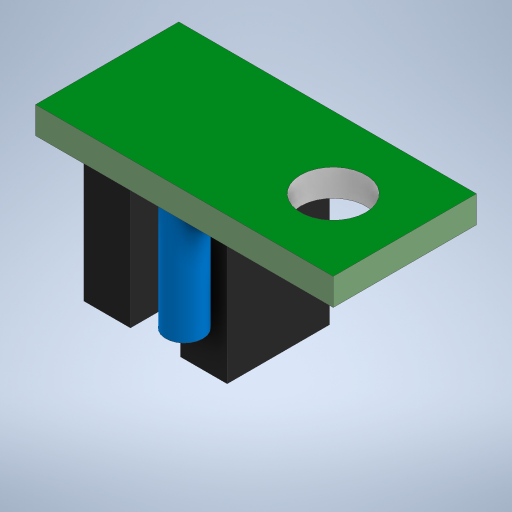
# Autodesk Inventor part: qre_module
Saved by Autodesk Inventor 2024 (Build 280153000, 153)
## iProperties
Created: 2023-11-08
Part Number: qre_module
Material: Všeobecné
Document SubType Name: Modeling
Designer: Simak
Density: 1 g/cm^3
Appearance: Výchozí
Author: Simak
Autodesk Inventor part; units mm, degrees
ref_plane "YZ Plane" through (0, 0, 0) normal (1, 0, 0) x (0, 1, 0)
ref_plane "XZ Plane" through (0, 0, 0) normal (0, 1, 0) x (-1, 0, 0)
ref_plane "XY Plane" through (0, 0, 0) normal (0, 0, 1) x (1, 0, 0)
sketch "Náčrt1" plane through (0, 0, 0) normal (0, 1, 0) x (-1, 0, 0)
  line L0 (8, -3.85) -> (-8, -3.85)
  line L1 (-8, -3.85) -> (-8, 3.85)
  line L2 (-8, 3.85) -> (8, 3.85)
  line L3 (8, 3.85) -> (8, -3.85)
  line L4 (8, -3.85) -> (0, 0) construction
  line L5 (8, 3.85) -> (0, 0) construction
  line L6 (-8, -3.85) -> (0, 0) construction
  dimension "d0" = 16
  dimension "d1" = 7.7
  constraints: 14 end point, 2 equal length, 2 parallel, 1 horizontal, 1 perpendicular
  measures "d0" distance of L0.start L0.end
  measures "d1" distance of L0.end L1.end
extrude "Vysunutí1" add sketch "Náčrt1" along normal blind 1.45
sketch "Náčrt2" plane through (0, 0, 0) normal (0, -1, 0) x (1, 0, 0)
  line L0 (0.2, 1.75) -> (-2.3, 1.75)
  line L1 (-2.3, 1.75) -> (-2.3, -3.75)
  line L2 (-2.3, -3.75) -> (0.2, -3.75)
  line L3 (0.2, -3.75) -> (0.2, 1.75)
  line L4 (-5, 1.75) -> (-7.5, 1.75)
  line L5 (-7.5, 1.75) -> (-7.5, -3.75)
  line L6 (-7.5, -3.75) -> (-5, -3.75)
  line L7 (-5, -3.75) -> (-5, 1.75)
  line L8 (-8, -3.85) -> (-8, 3.85) projected
  line L9 (-2.3, 1.75) -> (-5, 1.75) construction
  circle A0 centre (-3.65, -2.45) radius 1
  circle A1 centre (-1.05, 2.8) radius 1
  line L10 (-1.05, 1.75) -> (-1.05, 2.8) construction
  line L11 (-1.05, 2.8) -> (-1.05, 3.85) construction
  line L12 (-2.3, -2.45) -> (-3.65, -2.45) construction
  line L13 (-3.65, -2.45) -> (-5, -2.45) construction
  line L14 (-3.65, 1.75) -> (-3.65, 0.35) construction
  line L15 (-3.65, 0.35) -> (-3.65, -1.05) construction
  line L16 (-3.65, -1.05) -> (-3.65, -2.45) construction
  line L17 (-3.65, -3.85) -> (-3.65, -2.45) construction
  point P0 (0, 0)
  dimension "d4" = 2.5
  dimension "d5" = 5.5
  dimension "d6" = 0.5
  dimension "d7" = 2
  dimension "d8" = 2.7
  dimension "d15" = 0.1
  constraints: 34 end point, 8 point on line, 6 collinear, 5 equal length, 3 horizontal, 3 perpendicular, 2 centre point, 2 horizontal alignment, 2 midpoint, 2 vertical, 1 equal radius
  measures "d4" distance of L0.start L0.end
  measures "d5" distance of L2.end L0.start
  measures "d6" distance between parallel lines of L5 L8
  measures "d7" diameter of A0
  measures "d8" distance of L0.end L4.start
  measures "d15" vertical distance of L8.start L5.end
extrude "Vysunutí2" add sketch "Náčrt2" along normal blind 8.5 contours L3 L2 L1 L0 | L7 L6 L5 L4
extrude "Vysunutí3" add sketch "Náčrt2" along normal blind 6 contours A0 | A1
sketch "Náčrt3" plane through (0, 1.45, 0) normal (0, 1, 0) x (1, 0, 0)
  line L0 (8, -3.85) -> (8, 3.85) projected
  line L1 (8, -3.85) -> (4.15, -3.85)
  line L2 (4.15, -3.85) -> (4.15, 0)
  line L3 (4.15, 0) -> (8, 0)
  line L4 (8, 0) -> (8, -3.85)
  line L5 (8, 3.85) -> (-8, 3.85) projected
  line L6 (8, 3.85) -> (4.15, 3.85)
  line L7 (4.15, 3.85) -> (4.15, 0)
  line L8 (4.15, 0) -> (8, 0)
  line L9 (8, 0) -> (8, 3.85)
  point P0 (0, 0)
  constraints: 16 end point, 4 parallel, 4 perpendicular, 2 horizontal
hole "Díra1" at (4.15, 1.45, 0) direction (0, -1, 0) diameter 3.5 end through all
